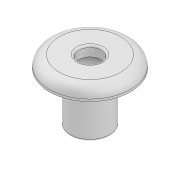
# Autodesk Inventor part: Remache POP Abierto con Rotura de Vástago D4
Saved by Autodesk Inventor 2020.3 (Build 243373000, 373)
## iProperties
Created: 2020-06-08
Part Number: Remache POP Abierto con Rotura de Vástago D4
Material: Aluminum 7175 T73 0 Hot Formed
Document SubType Name: Modeling
Designer: Dante
Density: 2.8 g/cm^3
Appearance: Satin
Author: Dante
Autodesk Inventor part; units mm, degrees
ref_plane "YZ Plane" through (0, 0, 0) normal (1, 0, 0) x (0, 1, 0)
ref_plane "XZ Plane" through (0, 0, 0) normal (0, 1, 0) x (-1, 0, 0)
ref_plane "XY Plane" through (0, 0, 0) normal (0, 0, 1) x (1, 0, 0)
sketch "Sketch1" plane through (0, 0, 0) normal (0, 0, 1) x (1, 0, 0)
  line L0 (-17.2279, 3.4821) -> (-17.2279, 3.7021)
  line L1 (-13.1179, 4.7021) -> (-16.2279, 4.7021)
  arc A0 (-16.2279, 4.7021) -> (-17.2279, 3.7021) centre (-16.2279, 3.7021) ccw
  line L2 (-15.1179, -1.5179) -> (-13.1179, -1.5179)
  line L3 (-15.1179, -1.5179) -> (-15.1179, 3.4821)
  line L4 (-13.1179, -1.5179) -> (-13.1179, 4.7021)
  line L5 (-17.2279, 3.4821) -> (-13.1179, 3.4821)
  point P0 (-17.2279, 4.7021)
  dimension "d0" = 1.22
  dimension "d2" = 1
  dimension "d7" = 2
  dimension "d8" = 3.11
  dimension "d9" = 4.11
  dimension "d10" = 6.22
  dimension "d11" = 5
  constraints: 12 end point, 4 point on line, 2 point on circle, 2 tangent, 1 centre point, 1 horizontal, 1 perpendicular, 1 vertical
  measures "d0" distance of L0.start point (-17.228, 4.702)
  measures "d2" radius of A0
  measures "d7" distance between parallel lines of L3 L4
  measures "d8" distance of L1.start L1.end
  measures "d9" distance of L0.start L5.end
  measures "d10" distance of L2.end L1.start
  measures "d11" distance of L2.start L3.end
revolve "Revolution1" add sketch "Sketch1" angle 360 about axis through (-13.1179, -1.5179, 0) along (0, 1, 0)
sketch "Sketch2" plane through (-13.1179, 4.7021, 0) normal (0, 1, 0) x (1, 0, 0)
  circle A0 centre (0, 0) radius 1.145
  dimension "d13" = 2.29
  constraints: 1 centre point
  measures "d13" diameter of A0
extrude "Extrusion1" cut sketch "Sketch2" against normal blind 10
fillet "Fillet1" radius 0.2 1 edges at (-14.2629, 4.7021, 0)
sketch "Sketch3" plane through (-13.1179, -1.5179, 0) normal (0, -1, 0) x (1, 0, 0)
  circle A0 centre (0, 0) radius 1.6
  dimension "d17" = 3.2
  constraints: 1 centre point
  measures "d17" diameter of A0
extrude "Extrusion2" cut sketch "Sketch3" against normal blind 5.2
fillet "Fillet2" radius 0.2 1 edges at (-14.7179, -1.5179, 0)
fillet "Fillet3" radius 0.2 1 edges at (-11.1179, -1.5179, 0)
body "Solid1"
